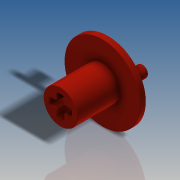
# Autodesk Inventor part: 99543-Red
Saved by Autodesk Inventor 2016 SP2 (Build 200236200, 236)
## iProperties
Created: 2015-09-01
Part Number: 99543-Red
Material: ABS Plastic
Document SubType Name: Modeling
Designer: D. Kohfeld
Density: 1.06 g/cm^3
Appearance: Red
Mass: 0.563647 g
Surface Area: 8.55312 cm^2
Volume: 0.531743 cm^3
Author: D. Kohfeld
Autodesk Inventor part; units mm, degrees
ref_plane "YZ Plane" through (0, 0, 0) normal (1, 0, 0) x (0, 1, 0)
ref_plane "XZ Plane" through (0, 0, 0) normal (0, 1, 0) x (-1, 0, 0)
ref_plane "XY Plane" through (0, 0, 0) normal (0, 0, 1) x (1, 0, 0)
sketch "Sketch2" plane through (0, 0, 0) normal (0, 1, 0) x (-1, 0, 0)
  line L0 (3.6, 0) -> (8, 0)
  line L1 (8, 0) -> (8, -1.2)
  line L2 (8, -1.2) -> (0, -1.2)
  line L3 (0, -1.2) -> (0, 8.8)
  line L4 (0, 8.8) -> (3.6, 8.8)
  line L5 (3.6, 8.8) -> (3.6, 0)
  point P0 (0, 0)
  dimension "d0" = 7.2
  dimension "d1" = 16
  dimension "d2" = 1.2
  dimension "d3" = 8.8
  constraints: 12 end point, 3 horizontal, 3 vertical, 1 horizontal alignment, 1 point on line
  measures "d0" diameter of L5 L3
  measures "d1" diameter of L1 L3
  measures "d2" distance between parallel lines of L0 L2
  measures "d3" distance between parallel lines of L4 L0
revolve "Revolution1" add sketch "Sketch2" angle 360 about axis through (0, 0, -1.2) along (0, 0, 1)
sketch "Sketch3" plane through (0, 0, 8.8) normal (0, 0, 1) x (1, 0, 0)
  circle A0 centre (0, 0) radius 3.6 projected
  circle A1 centre (0, 0) radius 2.4 construction
  line L0 (-0.8, 2.2627) -> (-0.8, 0.8)
  line L1 (-0.8, 0.8) -> (-2.2627, 0.8)
  line L2 (-2.2627, -0.8) -> (-0.8, -0.8)
  line L3 (-0.8, -0.8) -> (-0.8, -2.2627)
  line L4 (0.8, -2.2627) -> (0.8, -0.8)
  line L5 (0.8, -0.8) -> (2.2627, -0.8)
  line L6 (2.2627, 0.8) -> (0.8, 0.8)
  line L7 (0.8, 0.8) -> (0.8, 2.2627)
  arc A2 (0.8, 2.2627) -> (-0.8, 2.2627) centre (0, 0) ccw
  arc A3 (-2.2627, 0.8) -> (-2.2627, -0.8) centre (0, 0) ccw
  arc A4 (-0.8, -2.2627) -> (0.8, -2.2627) centre (0, 0) ccw
  arc A5 (2.2627, -0.8) -> (2.2627, 0.8) centre (0, 0) ccw
  dimension "d5" = 4.8
  dimension "d6" = 1.6
  constraints: 16 end point, 8 point on circle, 7 equal length, 4 centre point, 4 horizontal, 4 vertical, 1 coincident, 14 other
  measures "d6" distance between parallel lines of L7 L0
extrude "Extrusion1" cut sketch "Sketch3" against normal blind 8 contours A2 L7 L6 A5 L5 L4 A4 L3 L2 A3 L1 L0
sketch "Sketch4" plane through (0, 0, -1.2) normal (0, 0, -1) x (-1, 0, 0)
  circle A0 centre (0, 0) radius 8 projected
  circle A1 centre (-4.8497, 2.8) radius 1.2
  circle A2 centre (4.8497, 2.8) radius 1.2
  circle A3 centre (0, -5.6) radius 1.2
  circle A4 centre (0, 0) radius 5.6 construction
  line L0 (-4.8497, 2.8) -> (0, 0) construction
  line L1 (0, 0) -> (4.8497, 2.8) construction
  dimension "d9" = 120
  dimension "d10" = 2.4
  dimension "d11" = 11.2
  constraints: 4 centre point, 4 end point, 3 point on circle, 2 equal radius, 1 coincident, 1 horizontal alignment, 1 vertical alignment
  measures "d9" angle of L1 L0
  measures "d10" diameter of A2
  measures "d11" diameter of A4
extrude "Extrusion2" add sketch "Sketch4" along normal blind 2.4 contours A1 | A2 | A3
fillet "Fillet1" radius 0.1 6 edges at (3.6, 0, 8.8) (8, 0, 0) (8, 0, -1.2) (6.0497, 2.8, -3.6) (-3.6497, 2.8, -3.6) (1.2, -5.6, -3.6)
equation "\"d0\" = tlad"
equation "\"d1\" = 2 * lu"
equation "\"d5\" = tpd"
equation "\"d6\" = axlet"
equation "\"d7\" = lu"
equation "\"d14\" = lf"
equation "\"tlad\" = 7.2"
equation "\"lu\" = 8"
equation "\"tpd\" = 4.8"
equation "\"axlet\" = 1.6"
equation "\"lf\" = 0.1"
body "Solid1"
